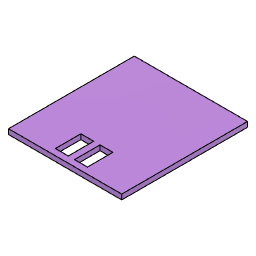
Post it Plotter v2 (Autodesk Fusion 360 archive; units mm, degrees)
design "base"
Autodesk Fusion 360 part; units mm, degrees
sketch "Skizze1" plane through (0, 0, 0) normal (0, 1, 0) x (1, 0, 0)
  line L0 (90, 100) -> (-90, 100)
  line L1 (-90, 100) -> (-90, -100)
  line L2 (-90, -100) -> (90, -100)
  line L3 (90, -100) -> (90, 100)
  line L4 (90, 100) -> (-90, -100) construction
  line L5 (-90, 100) -> (90, -100) construction
  line L6 (-5, -49.5) -> (-25.5, -49.5)
  line L7 (-25.5, -49.5) -> (-25.5, -90)
  line L8 (-25.5, -90) -> (-5, -90)
  line L9 (-5, -90) -> (-5, -49.5)
  line L10 (-5, -49.5) -> (-25.5, -90) construction
  line L11 (-25.5, -49.5) -> (-5, -90) construction
  line L12 (0, 100) -> (0, -100)
  line L13 (25.5, -49.5) -> (25.5, -90)
  line L14 (25.5, -90) -> (5, -90)
  line L15 (5, -49.5) -> (25.5, -49.5)
  line L16 (5, -90) -> (5, -49.5)
  point P0 (-15.25, -69.75)
  dimension "d1" = 180
  dimension "d2" = 200
  dimension "d5" = 20.5
  dimension "d6" = 40.5
  dimension "d7" = 5
  dimension "d9" = 10
  constraint horizontal L0
  constraint perpendicular L0 L1
  constraint parallel L0 L2
  constraint parallel L1 L3
  constraint coincident L4 origin
  constraint coincident L5 origin
  constraint horizontal L6
  constraint perpendicular L6 L7
  constraint parallel L6 L8
  constraint parallel L7 L9
  constraint coincident L10 P0
  constraint coincident L11 P0
  constraint midpoint L0 L12.start
  constraint midpoint L2 L12.end
  constraint symmetric L6.start L12 L15.start
  constraint symmetric L6.end L12 L13.start
  constraint symmetric L7.end L12 L13.end
  constraint symmetric L8.end L12 L14.end
  measures "d1" distance of L1.end L2.end
  measures "d2" distance of L0.end L1.end
  measures "d5" distance of L7.end L8.end
  measures "d6" distance of L6.end L7.end
  measures "d7" distance of origin L9
  measures "d9" distance of L2 L8
extrude "Extrusion1" add sketch "Skizze1" against normal blind 8 makes body 1
copy_body "Körper->Berechn1" bodies 1 removing the originals makes body 2 in component "base"
component "base" placed x (1, 0, 0) y (0, 1, 0) z (0, 0, 1) at (0, 0, 0)
named bodies: "base"

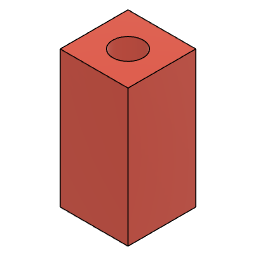
design "foot"
Autodesk Fusion 360 part; units mm, degrees
sketch "Skizze1" plane through (0, 0, 0) normal (0, 1, 0) x (1, 0, 0)
  line L0 (5, 5) -> (-5, 5)
  line L1 (-5, 5) -> (-5, -5)
  line L2 (-5, -5) -> (5, -5)
  line L3 (5, -5) -> (5, 5)
  line L4 (5, 5) -> (-5, -5) construction
  line L5 (-5, 5) -> (5, -5) construction
  dimension "d1" = 10
  dimension "d2" = 10
  constraint horizontal L0
  constraint perpendicular L0 L1
  constraint parallel L0 L2
  constraint parallel L1 L3
  constraint coincident L4 origin
  constraint coincident L5 origin
  measures "d1" distance of L1.end L2.end
  measures "d2" distance of L0.end L1.end
extrude "Extrusion1" add sketch "Skizze1" along normal blind 20.2 makes body 1
copy_body "Körper->Berechn1" bodies 1 removing the originals makes body 2 in component "foot"
hole "Bohrung1" at (0, 20.2, 0) direction (0, -1, 0) diameter 4.5 depth 10 tip angle 118 bodies 2 in component "foot"
component "foot" placed x (1, 0, 0) y (0, 1, 0) z (0, 0, 1) at (0, 0, 0)
named bodies: "foot"

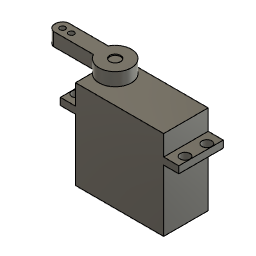
design "servo DS3218"
Autodesk Fusion 360 part; units mm, degrees
sketch "Skizze1" plane through (0, 0, 0) normal (0, 1, 0) x (1, 0, 0)
  line L0 (20.2, 10.2) -> (-20.2, 10.2)
  line L1 (-20.2, 10.2) -> (-20.2, -10.2)
  line L2 (-20.2, -10.2) -> (20.2, -10.2)
  line L3 (20.2, -10.2) -> (20.2, 10.2)
  line L4 (20.2, 10.2) -> (-20.2, -10.2) construction
  line L5 (-20.2, 10.2) -> (20.2, -10.2) construction
  line L6 (-27.15, -10.2) -> (27.15, -10.2)
  line L7 (27.15, -10.2) -> (27.15, 10.2)
  line L8 (27.15, 10.2) -> (-27.15, 10.2)
  line L9 (-27.15, 10.2) -> (-27.15, -10.2)
  line L10 (-27.15, -10.2) -> (27.15, 10.2) construction
  line L11 (27.15, -10.2) -> (-27.15, 10.2) construction
  line L12 (-24.8, -5) -> (24.8, -5)
  line L13 (24.8, -5) -> (24.8, 5)
  line L14 (24.8, 5) -> (-24.8, 5)
  line L15 (-24.8, 5) -> (-24.8, -5)
  line L16 (-24.8, -5) -> (24.8, 5) construction
  line L17 (24.8, -5) -> (-24.8, 5) construction
  circle A0 centre (24.8, 5) radius 2.25
  circle A1 centre (24.8, -5) radius 2.25
  circle A2 centre (-24.8, -5) radius 2.25
  circle A3 centre (-24.8, 5) radius 2.25
  dimension "d1" = 40.4
  dimension "d2" = 20.4
  dimension "d5" = 54.3
  dimension "d6" = 49.6
  dimension "d7" = 10
  dimension "d8" = 4.5
  dimension "d9" = 4.5
  dimension "d10" = 4.5
  dimension "d11" = 4.5
  constraint horizontal L0
  constraint perpendicular L0 L1
  constraint parallel L0 L2
  constraint parallel L1 L3
  constraint coincident L4 origin
  constraint coincident L5 origin
  constraint horizontal L6
  constraint perpendicular L6 L7
  constraint parallel L6 L8
  constraint parallel L7 L9
  constraint coincident L10 origin
  constraint coincident L11 origin
  constraint horizontal L12
  constraint perpendicular L12 L13
  constraint parallel L12 L14
  constraint parallel L13 L15
  constraint coincident L16 origin
  constraint coincident L17 origin
  constraint coincident L13.end L14.start
  constraint coincident L12.end L13.start
  constraint coincident L12.start L15.end
  constraint coincident L14.end L15.start
  measures "d1" distance of L1.end L2.end
  measures "d2" distance of L0.end L1.end
  measures "d5" distance of L7.end L8.end
  measures "d6" distance of L13.end L14.end
  measures "d7" distance of L12.end L13.end
  measures "d8" diameter of A0
  measures "d9" diameter of A1
  measures "d10" diameter of A2
  measures "d11" diameter of A3
extrude "Extrusion1" add sketch "Skizze1" against normal blind 28.3 contours L0 L1 L3 L8 L14 | L1 L3 L12 L14 | L1 L2 L3 L6 L12 makes body 1
extrude "Extrusion2" add sketch "Skizze1" along normal blind 3.2 contours L0 L1 L3 L8 L14 | L3 L6 L7 L8 L12 L13 L14 A0 A1 | L1 L6 L8 L9 L12 L14 L15 A2 A3 | L3 L12 L13 L14 A0 A1 | L1 L3 L12 L14 | L1 L12 L14 L15 A2 A3 | L1 L2 L3 L6 L12 bodies 1
extrude "Extrusion3" add sketch "Skizze1" along normal blind 12.5 contours L0 L1 L3 L8 L14 | L1 L3 L12 L14 | L1 L2 L3 L6 L12 bodies 1
sketch "Skizze2" plane through (0, 12.5, 0) normal (0, 1, 0) x (-1, 0, 0)
  line L0 (-20.2, 10.2) -> (-20.2, -10.2)
  line L1 (-20.2, -10.2) -> (20.2, -10.2)
  line L2 (20.2, -10.2) -> (20.2, 10.2)
  line L3 (20.2, 10.2) -> (-20.2, 10.2)
  circle A0 centre (12.2, 0) radius 2.5
  dimension "d16" = 5
  dimension "d17" = 8
  measures "d16" diameter of A0
  measures "d17" distance of L2 A0.centre
extrude "Extrusion4" add sketch "Skizze2" along normal blind 8 contours A0 bodies 1
sketch "Skizze3" plane through (0, 20.5, 0) normal (0, 1, 0) x (-1, 0, 0)
  circle A0 centre (12.2, 0) radius 2.5
  circle A1 centre (12.2, 0) radius 7.4
  line L0 (12.2, -3.4) -> (39.8, -3.4)
  line L1 (39.8, -3.4) -> (39.8, 3.4)
  line L2 (39.8, 3.4) -> (12.2, 3.4)
  line L3 (12.2, 3.4) -> (12.2, -3.4)
  line L4 (12.2, -3.4) -> (39.8, 3.4) construction
  line L5 (39.8, -3.4) -> (12.2, 3.4) construction
  circle A2 centre (32.3, 0) radius 1.25
  circle A3 centre (36.3, 0) radius 1.25
  circle A4 centre (36.3, 0) radius 3.5005
  line L6 (39.8, 0) -> (12.2, 0)
  point P0 (26, 0)
  dimension "d20" = 14.8
  dimension "d21" = 27.6
  dimension "d22" = 6.8
  dimension "d23" = 2.5
  dimension "d24" = 2.5
  dimension "d25" = 7.5
  dimension "d26" = 3.5
  constraint concentric A0 A1
  constraint horizontal L0
  constraint perpendicular L0 L1
  constraint parallel L0 L2
  constraint parallel L1 L3
  constraint coincident L4 P0
  constraint coincident L5 P0
  constraint coincident A0.centre L3
  constraint concentric A3 A4
  constraint midpoint L1 L6.start
  constraint midpoint L3 A0.centre
  constraint coincident A0.centre A1.centre
  constraint coincident A3.centre L6
  constraint coincident A2.centre L6
  measures "d20" diameter of A1
  measures "d21" distance of A0.centre L1
  measures "d22" distance of L0 L2
  measures "d23" diameter of A2
  measures "d24" diameter of A3
  measures "d25" distance of L1 A2.centre
  measures "d26" distance of L1 A3.centre
extrude "Extrusion5" add sketch "Skizze3" along normal blind 6 separate body contours A0 A1 L0 L3 L6 | A0 A1 L2 L3 L6 | A0 A1 L0 L2 L3 | A1 L0 A2 A4 L6 | A1 L2 A2 A4 L6 | L2 A2 A3 A4 L6 | L0 A2 A3 A4 L6 makes body 2
move_body "Verschieben1" bodies 2 to x (1, 0, 0) y (0, 1, 0) z (0, 0, 1) at (0, -5.5, 0)
copy_body "Körper->Berechn1" bodies 1 removing the originals makes body 3 in component "servo"
copy_body "Körper->Berechn2" bodies 2 removing the originals makes body 4 in component "servo arm"
component "servo" placed x (1, 0, 0) y (0, 1, 0) z (0, 0, 1) at (0, 0, 0)
component "servo arm" placed x (1, 0, 0) y (0, 1, 0) z (0, 0, 1) at (0, 0, 0)
equation "d21 = 35 mm - 7.4 mm"
named bodies: "servo", "servo arm"

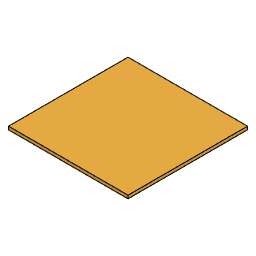
design "Post It"
Autodesk Fusion 360 part; units mm, degrees
sketch "Skizze1" plane through (0, 0, 0) normal (0, 1, 0) x (1, 0, 0)
  line L0 (38.1, 38.1) -> (-38.1, 38.1)
  line L1 (-38.1, 38.1) -> (-38.1, -38.1)
  line L2 (-38.1, -38.1) -> (38.1, -38.1)
  line L3 (38.1, -38.1) -> (38.1, 38.1)
  line L4 (38.1, 38.1) -> (-38.1, -38.1) construction
  line L5 (-38.1, 38.1) -> (38.1, -38.1) construction
  dimension "d1" = 76.2
  dimension "d2" = 76.2
  constraint perpendicular L0 L1
  constraint parallel L0 L2
  constraint parallel L1 L3
  constraint horizontal L0
  constraint coincident L4 origin
  constraint coincident L5 origin
  measures "d1" distance of L1.end L2.end
  measures "d2" distance of L0.end L1.end
extrude "Extrusion1" add sketch "Skizze1" along normal blind 2 makes body 1
copy_body "Körper->Berechn1" bodies 1 removing the originals makes body 2 in component "Post It"
component "Post It" placed x (1, 0, 0) y (0, 1, 0) z (0, 0, 1) at (0, 0, 0)
named bodies: "Post It"

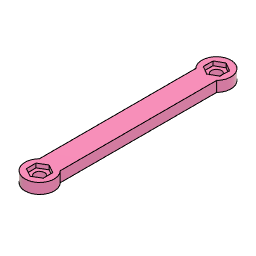
design "right arm"
Autodesk Fusion 360 part; units mm, degrees
sketch "Skizze1" plane through (0, 0, 0) normal (0, 1, 0) x (1, 0, 0)
  circle A0 centre (20, -96) radius 2.4
  circle A1 centre (20, -96) radius 3.5
  circle A2 centre (20, -96) radius 5
  line L0 (25, -96) -> (15, -96)
  line L1 (15, -96) -> (15, -11)
  line L2 (15, -11) -> (25, -11)
  line L3 (25, -11) -> (25, -96)
  line L4 (25, -96) -> (15, -11) construction
  line L5 (15, -96) -> (25, -11) construction
  line L6 (15, -53.5) -> (25, -53.5)
  line L7 (16.0244, -98.3512) -> (20.0484, -100.6185)
  line L8 (20.0484, -100.6185) -> (24.024, -98.2673)
  line L9 (24.024, -98.2673) -> (23.9756, -93.6488)
  line L10 (23.9756, -93.6488) -> (19.9516, -91.3815)
  line L11 (19.9516, -91.3815) -> (15.976, -93.7327)
  line L12 (15.976, -93.7327) -> (16.0244, -98.3512)
  circle A3 centre (20, -96) radius 7
  circle A4 centre (20, -96) radius 9
  circle A5 centre (20, -11) radius 9
  circle A6 centre (20, -11) radius 7
  line L13 (19.9516, -15.6185) -> (15.976, -13.2673)
  line L14 (15.976, -13.2673) -> (16.0244, -8.6488)
  line L15 (16.0244, -8.6488) -> (20.0484, -6.3815)
  line L16 (20.0484, -6.3815) -> (24.024, -8.7327)
  line L17 (23.9756, -13.3512) -> (19.9516, -15.6185)
  line L18 (24.024, -8.7327) -> (23.9756, -13.3512)
  circle A7 centre (20, -11) radius 5
  circle A8 centre (20, -11) radius 3.5
  circle A9 centre (20, -11) radius 2.4
  line L19 (20, -96) -> (26.4279, -103.6604)
  line L20 (20, -96) -> (40, -96) construction
  line L21 (16.2945, -99.3569) -> (22.6004, -106.8721)
  line L22 (22.6004, -106.8721) -> (30.2553, -100.4488)
  line L23 (30.2553, -100.4488) -> (23.9494, -92.9337)
  point P0 (20, -53.5)
  point P1 (20, -96)
  dimension "d1" = 4.8
  dimension "d2" = 7
  dimension "d3" = 10
  dimension "d5" = 4
  dimension "d6" = 14
  dimension "d7" = 18
  dimension "d18" = 50
  dimension "d19" = 10
  dimension "d22" = 85
  dimension "d23" = 10
  constraint concentric A0 A1
  constraint concentric A0 A2
  constraint horizontal L0
  constraint perpendicular L0 L1
  constraint parallel L0 L2
  constraint parallel L1 L3
  constraint coincident L4 P0
  constraint coincident L5 P0
  constraint coincident A2 L0.start
  constraint coincident A2 L0.end
  constraint midpoint L1 L6.start
  constraint midpoint L3 L6.end
  constraint coincident P1 A0.centre
  constraint concentric A0 A4
  constraint symmetric A0 L6 A9
  constraint symmetric A1 L6 A8
  constraint symmetric A2 L6 A7
  constraint symmetric L6 L7.start L14.end
  constraint symmetric L6 L7.end L15.end
  constraint symmetric L6 L8.end L16.end
  constraint symmetric L6 L9.end L17.start
  constraint symmetric L6 L10.end L13.start
  constraint symmetric L6 L11.end L13.end
  constraint symmetric L6 A3 A6
  constraint symmetric L6 A4 A5
  constraint horizontal L20
  constraint coincident A2 L21.start
  constraint coincident A2 L23.end
  constraint coincident L19.end L22
  constraint midpoint L19.end L22
  constraint perpendicular L22 L23
  constraint perpendicular L21 L22
  constraint parallel L19 L21
  measures "d1" diameter of A0
  measures "d2" diameter of A1
  measures "d3" diameter of A2
  measures "d5" distance of P1 L12
  measures "d6" diameter of A3
  measures "d7" diameter of A4
  measures "d18" angle of L19 L20
  measures "d19" distance of P1 L19.end
  measures "d22" distance of P1 A5.centre
  measures "d23" distance of L1 L3
extrude "Extrusion1" add sketch "Skizze1" along normal blind 2 contours A2 L0 L9 L10 L11 L12 | A2 L0 L8 L9 L19 | A2 L0 L7 L8 L12 L19 | A2 L3 A3 L19 L23 | A2 L3 L23 | A2 L1 L3 A3 L23 | A2 L1 A3 L21 | A2 A3 L19 L21 | L3 A3 L23 | L1 L3 A3 A4 | L1 L3 L6 A4 | L1 L3 L6 A5 | L1 L3 A5 A6 | L1 L3 A6 A7 | L1 L3 A6 A7 | L2 L14 L15 L16 L18 A7 | L2 L13 L14 L17 L18 A7 picked at (20.6088, -19.2948)
extrude "Extrusion2" add sketch "Skizze1" against normal blind 3 contours A1 L0 L8 L9 L19 | A1 L0 L9 L10 L11 L12 | A1 L0 L7 L8 L12 L19 | A2 L0 L9 L10 L11 L12 | A2 L0 L8 L9 L19 | A2 L0 L7 L8 L12 L19 | A2 L3 A3 L19 L23 | A2 L3 L23 | A2 L1 L3 A3 L23 | A2 L1 A3 L21 | A2 A3 L19 L21 | L3 A3 L23 | L1 L3 A3 A4 | L1 L3 L6 A4 | L1 L3 L6 A5 | L1 L3 A5 A6 | L1 L3 A6 A7 | L1 L3 A6 A7 | L2 L14 L15 L16 L18 A7 | L2 L13 L14 L17 L18 A7 | L2 L14 L15 L16 L18 A8 | L2 L13 L14 L17 L18 A8 picked at (20.6088, -19.2948)
extrude "Extrusion3" add sketch "Skizze1" against normal blind 5 contours A0 A1 L0 L19 | A0 A1 L0 | A0 A1 L0 L19 | L2 A8 A9 | L2 A8 A9
chamfer "Fase1" distance 2 angle 45 2 edges at (16.7369, -3, 97.2657) (16.7369, -3, 12.2657)
extrude "Extrusion8" [rolled back] along distance 2 taper angle 0 against distance 3 side2taper angle 0
sketch "Skizze2" plane through (0, 2, 0) normal (0, 1, 0) x (-1, 0, 0)
  line L0 (-16.0244, 98.3512) -> (-15.976, 93.7327)
  line L1 (-15.976, 93.7327) -> (-19.9516, 91.3815)
  line L2 (-19.9516, 91.3815) -> (-23.9756, 93.6488)
  line L3 (-23.9756, 93.6488) -> (-24.024, 98.2673)
  line L4 (-24.024, 98.2673) -> (-20.0484, 100.6185)
  line L5 (-20.0484, 100.6185) -> (-16.0244, 98.3512)
  line L6 (-20.0484, 6.3815) -> (-24.024, 8.7327)
  line L7 (-24.024, 8.7327) -> (-23.9756, 13.3512)
  line L8 (-23.9756, 13.3512) -> (-19.9516, 15.6185)
  line L9 (-19.9516, 15.6185) -> (-15.976, 13.2673)
  line L10 (-15.976, 13.2673) -> (-16.0244, 8.6488)
  line L11 (-16.0244, 8.6488) -> (-20.0484, 6.3815)
  arc A0 (-15, 91.101) -> (-19.3239, 102.9673) centre (-20, 96) ccw
  line L12 (-19.3239, 102.9673) -> (-22.6004, 106.8721)
  line L13 (-22.6004, 106.8721) -> (-30.2553, 100.4488)
  line L14 (-30.2553, 100.4488) -> (-26.9788, 96.544)
  arc A1 (-26.9788, 96.544) -> (-25, 91.101) centre (-20, 96) ccw
  line L15 (-25, 91.101) -> (-25, 15.899)
  arc A2 (-25, 15.899) -> (-15, 15.899) centre (-20, 11) ccw
  line L16 (-15, 15.899) -> (-15, 91.101)
  line L17 (-25.3367, 106.0773) -> (-26.1087, 110.4553)
  line L18 (-26.1087, 110.4553) -> (-30.2862, 111.9758)
  line L19 (-30.2862, 111.9758) -> (-33.6917, 109.1182)
  line L20 (-33.6917, 109.1182) -> (-32.9197, 104.7402)
  line L21 (-32.9197, 104.7402) -> (-28.7422, 103.2197)
  line L22 (-28.7422, 103.2197) -> (-25.3367, 106.0773)
  line L23 (-24.9569, 105.939) -> (-25.7991, 110.7151)
  line L24 (-25.7991, 110.7151) -> (-30.3563, 112.3738)
  line L25 (-30.3563, 112.3738) -> (-34.0715, 109.2565)
  line L26 (-34.0715, 109.2565) -> (-33.2293, 104.4804)
  line L27 (-33.2293, 104.4804) -> (-28.672, 102.8217)
  line L28 (-28.672, 102.8217) -> (-24.9569, 105.939)
  line L29 (-22.6004, 106.8721) -> (-30.2553, 100.4488)
  circle A3 centre (-29.5142, 107.5978) radius 6
  line L30 (-30.2553, 100.4488) -> (-31.5045, 101.9375)
  line L31 (-22.6004, 106.8721) -> (-23.5261, 107.9752)
  line L32 (-24.3181, 105.6688) -> (-25.2456, 111.1332)
  line L33 (-25.2456, 111.1332) -> (-30.4417, 113.0622)
  line L34 (-30.4417, 113.0622) -> (-34.7103, 109.5267)
  line L35 (-34.7103, 109.5267) -> (-33.7828, 104.0623)
  line L36 (-33.7828, 104.0623) -> (-28.5867, 102.1333)
  line L37 (-28.5867, 102.1333) -> (-24.3181, 105.6688)
  point P0 (-29.5142, 107.5978)
  point P1 (-29.5142, 107.5978)
  point P2 (-29.5142, 107.5978)
  dimension "d24" = 3.85
  dimension "d25" = 4.2
  dimension "d26" = 12
  dimension "d27" = 5
  dimension "d30" = 4.8
  constraint coincident P2 P1
  constraint parallel L28 L29
  constraint parallel L22 L28
  constraint coincident L13.end L14.start
  constraint coincident A3 L30.end
  constraint perpendicular L29 L30
  constraint coincident L12.end L13.start
  constraint coincident A3 L31.end
  constraint perpendicular L13 L31
  measures "d24" distance of P2 L22
  measures "d25" distance of P2 L28
  measures "d26" diameter of A3
  measures "d27" distance of P2 L29
  measures "d30" distance of P2 L37
extrude "Extrusion6" [rolled back] along distance -5 taper angle 0
extrude "Extrusion7" [rolled back] along distance -40 taper angle 0
equation "d24 = ( 7.7 / 2 ) * 1 mm"
named bodies: "left arm"

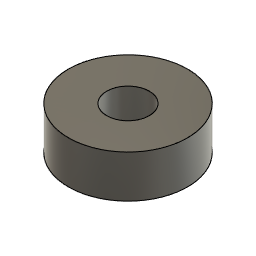
design "bearing"
Autodesk Fusion 360 part; units mm, degrees
sketch "Skizze1" plane through (0, 0, 0) normal (0, 1, 0) x (1, 0, 0)
  circle A0 centre (0, 0) radius 7
  circle A1 centre (0, 0) radius 2.5
  dimension "d1" = 14
  dimension "d2" = 5
  constraint coincident A0.centre A1.centre
  constraint concentric A0 A1
  measures "d1" diameter of A0
  measures "d2" diameter of A1
extrude "Extrusion1" add sketch "Skizze1" along normal blind 5 makes body 1
copy_body "Körper->Berechn1" bodies 1 removing the originals makes body 2 in component "bearing"
component "bearing" placed x (1, 0, 0) y (0, 1, 0) z (0, 0, 1) at (0, 0, 0)
named bodies: "bearing"

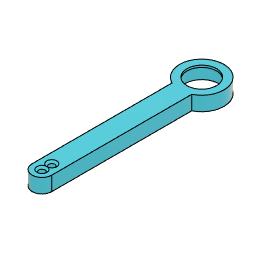
design "near arm"
Autodesk Fusion 360 part; units mm, degrees
sketch "Skizze1" plane through (0, 0, 0) normal (0, 1, 0) x (1, 0, 0)
  line L0 (4, 35) -> (-4, 35)
  line L1 (-4, 35) -> (-4, -35)
  line L2 (-4, -35) -> (4, -35)
  line L3 (4, -35) -> (4, 35)
  line L4 (4, 35) -> (-4, -35) construction
  line L5 (-4, 35) -> (4, -35) construction
  circle A0 centre (0, -30) radius 1.25
  circle A1 centre (0.0004, -26) radius 1.25
  circle A2 centre (0, 34.9) radius 9
  circle A3 centre (0, 34.9) radius 7
  circle A4 centre (0, -30) radius 4
  line L6 (0, 35) -> (0, -35)
  circle A5 centre (0, 34.9) radius 6
  dimension "d1" = 8
  dimension "d2" = 70
  dimension "d3" = 2.5
  dimension "d4" = 2.5
  dimension "d5" = 4
  dimension "d6" = 5
  dimension "d7" = 18
  dimension "d8" = 14
  dimension "d9" = 64.9
  dimension "d12" = 12
  constraint horizontal L0
  constraint perpendicular L0 L1
  constraint parallel L0 L2
  constraint parallel L1 L3
  constraint coincident L4 origin
  constraint coincident L5 origin
  constraint concentric A2 A3
  constraint concentric A0 A4
  constraint tangent L3 A4
  constraint midpoint L0 L6.start
  constraint midpoint L2 L6.end
  constraint coincident A0.centre L6
  constraint coincident A2.centre L6
  constraint concentric A2 A5
  measures "d1" distance of L1.end L2.end
  measures "d2" distance of L0.end L1.end
  measures "d3" diameter of A0
  measures "d4" diameter of A1
  measures "d5" distance of A0.centre A1.centre
  measures "d6" distance of L2 A0.centre
  measures "d7" diameter of A2
  measures "d8" diameter of A3
  measures "d9" distance of A0.centre A2.centre
  measures "d12" diameter of A5
extrude "Extrusion1" add sketch "Skizze1" against normal blind 5 contours L1 L3 A2 A3 | L3 A2 A3 L6 | L1 A2 A3 L6 | L3 A1 A2 A4 L6 | L1 A1 A2 A4 L6 | A0 A1 A4 L6 | A0 A1 A4 L6 makes body 1
extrude "Extrusion2" add sketch "Skizze1" along normal blind 0.8 contours L1 L3 A3 A5 | L3 A3 L6 A5 | L1 A3 L6 A5 | L1 L3 A2 A3 | L3 A2 A3 L6 | L1 A2 A3 L6 | L3 A1 A2 A4 L6 | L1 A1 A2 A4 L6 | A0 A1 A4 L6 | A0 A1 A4 L6 bodies 1
chamfer "Fase1" distance 0.8 angle 45 2 edges at (-1.165, 0.8, 25.548) (-1.1654, 0.8, 29.548) on bodies 1
copy_body "Körper->Berechn1" bodies 1 removing the originals makes body 2 in component "near arm"
component "near arm" placed x (1, 0, 0) y (0, 1, 0) z (0, 0, 1) at (0, 0, 0)
named bodies: "near arm"
